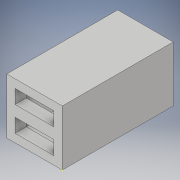
# Autodesk Inventor part: sensor pod
Saved by Autodesk Inventor 2018 (Build 220112000, 112)
## iProperties
Created: 2018-03-12
Part Number: sensor pod
Material: Generic
Document SubType Name: Modeling
Designer: Josh
Density: 1 g/cm^3
Appearance: Default
Author: Josh
Autodesk Inventor part; units mm, degrees
ref_plane "YZ Plane" through (0, 0, 0) normal (1, 0, 0) x (0, 1, 0)
ref_plane "XZ Plane" through (0, 0, 0) normal (0, 1, 0) x (-1, 0, 0)
sketch "Sketch1" plane through (0, 0, 0) normal (0, 1, 0) x (-1, 0, 0)
  point P0 (0, 0)
sketch "Sketch2" plane through (0, 0, 0) normal (0, 1, 0) x (-1, 0, 0)
  line L0 (0, 0) -> (25.4, 0)
  line L1 (25.4, 0) -> (25.4, -50.8)
  line L2 (25.4, -50.8) -> (0, -50.8)
  line L3 (0, -50.8) -> (0, 0)
  dimension "d0" = 25.4
  dimension "d1" = 50.8
  constraints: 8 end point, 2 parallel, 1 horizontal, 1 perpendicular
  measures "d0" distance of L1.end L2.end
  measures "d1" distance of L0.end L1.end
extrude "Extrusion1" add sketch "Sketch2" along normal blind 25.4
sketch "Sketch3" plane through (-25.4, 0, 0) normal (0, 0, 1) x (1, 0, 0)
  line L0 (0, 25.4) -> (25.4, 25.4) projected
  line L1 (0, 0) -> (0, 25.4) projected
  line L2 (25.4, 0) -> (25.4, 25.4) projected
  line L3 (3.81, 21.59) -> (21.59, 21.59)
  line L4 (21.59, 21.59) -> (21.59, 15.24)
  line L5 (21.59, 15.24) -> (3.81, 15.24)
  line L6 (3.81, 15.24) -> (3.81, 21.59)
  line L7 (25.4, 0) -> (0, 0) projected
  line L8 (3.81, 3.81) -> (21.59, 3.81)
  line L9 (21.59, 3.81) -> (21.59, 10.16)
  line L10 (21.59, 10.16) -> (3.81, 10.16)
  line L11 (3.81, 10.16) -> (3.81, 3.81)
  dimension "d4" = 3.81
  dimension "d5" = 3.81
  dimension "d6" = 3.81
  dimension "d7" = 6.35
  dimension "d8" = 3.81
  dimension "d9" = 6.35
  constraints: 16 end point, 4 parallel, 2 horizontal, 2 perpendicular
  measures "d4" distance from line of L0 L3.start
  measures "d5" distance from line of L1 L3.start
  measures "d6" distance from line of L2 point (21.59, 21.59)
  measures "d7" distance of L3.end L4.end
  measures "d8" distance from line of L7 L8.start
  measures "d9" distance of L9.end L8.end
extrude "Extrusion2" cut sketch "Sketch3" against normal blind 5.08 contours L3 L4 L5 L6 | L11 L10 L9 L8
ref_plane "Work Plane1" through (-25.4, 0, -5.08) normal (0, 0, 1) x (1, 0, 0)
sketch "Sketch4" plane through (-25.4, 0, -5.08) normal (0, 0, 1) x (1, 0, 0)
  line L0 (2.54, 22.86) -> (22.86, 22.86)
  line L1 (22.86, 22.86) -> (22.86, 2.54)
  line L2 (22.86, 2.54) -> (2.54, 2.54)
  line L3 (2.54, 2.54) -> (2.54, 22.86)
  line L4 (0, 25.4) -> (25.4, 25.4) projected
  line L5 (0, 0) -> (0, 25.4) projected
  line L6 (25.4, 0) -> (25.4, 25.4) projected
  line L7 (25.4, 0) -> (0, 0) projected
  dimension "d13" = 2.54
  dimension "d14" = 2.54
  dimension "d15" = 2.54
  dimension "d16" = 2.54
  constraints: 8 end point, 2 parallel, 1 horizontal, 1 perpendicular
  measures "d13" distance between parallel lines of L4 L0
  measures "d14" distance between parallel lines of L5 L3
  measures "d15" distance between parallel lines of L6 L1
  measures "d16" distance between parallel lines of L7 L2
extrude "Extrusion3" cut sketch "Sketch4" against normal blind 43.18 contours L0 L1 L2 L3
sketch "Sketch5" plane through (0, 0, -50.8) normal (0, 0, -1) x (-1, 0, 0)
  line L0 (2.54, 2.54) -> (22.86, 2.54) projected
  line L1 (9.525, 8.89) -> (15.875, 8.89)
  line L2 (15.875, 8.89) -> (15.875, 2.54)
  line L3 (15.875, 2.54) -> (9.525, 2.54)
  line L4 (9.525, 2.54) -> (9.525, 8.89)
  line L5 (0, 0) -> (0, 25.4) projected
  dimension "d19" = 6.35
  dimension "d20" = 6.35
  dimension "d21" = 9.525
  constraints: 8 end point, 2 parallel, 1 horizontal, 1 perpendicular, 1 point on line
  measures "d19" distance of L1.start L1.end
  measures "d20" distance of L3.end L1.start
  measures "d21" distance between parallel lines of L5 L4
extrude "Extrusion4" cut sketch "Sketch5" against normal blind 12.7
sketch "Sketch6" plane through (-22.86, 2.54, -5.08) normal (1, 0, 0) x (0, 0, -1)
  line L0 (15.6891, 18.5897) -> (25.8491, 18.5897)
  line L1 (25.8491, 18.5897) -> (25.8491, 8.4297)
  line L2 (25.8491, 8.4297) -> (15.6891, 8.4297)
  line L3 (15.6891, 8.4297) -> (15.6891, 18.5897)
  point P0 (-5.08, -2.54)
  dimension "d24" = 10.16
  dimension "d25" = 10.16
  constraints: 8 end point, 2 parallel, 1 horizontal, 1 perpendicular
  measures "d24" distance of L1.end L2.end
  measures "d25" distance of L0.end L1.end
extrude "Extrusion5" add sketch "Sketch6" along normal blind 5.08
sketch "Sketch7" plane through (-25.4, 0, -48.26) normal (0, 0, 1) x (1, 0, 0)
  line L0 (22.86, 2.54) -> (15.875, 2.54) projected
  line L1 (22.86, 22.86) -> (22.86, 2.54) projected
  circle A0 centre (19.8628, 5.54) radius 3
  point P0 (25.4, 0)
  dimension "d28" = 3
  dimension "d29" = 2.9972
  dimension "d30" = 6
  constraints: 1 centre point, 1 coincident
  measures "d28" distance from line of L0 point (19.863, 5.54)
  measures "d29" distance from line of L1 point (19.863, 5.54)
  measures "d30" diameter of A0
extrude "Extrusion6" add sketch "Sketch7" along normal blind 33.02 contours A0 L1 | L1 A0
body "Solid1"
